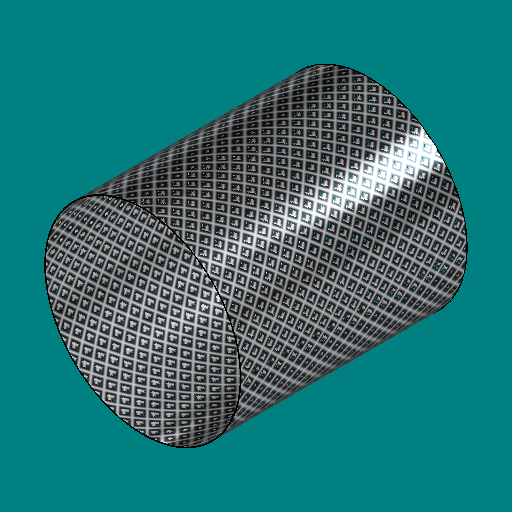
# Autodesk Inventor part: probe-port-mesh
Saved by Autodesk Inventor 2025 (Build 290162000, 162)
## iProperties
Created: 2024-06-28
Part Number: probe-port-mesh
Material: Stainless Steel
Document SubType Name: Modeling
Designer: kuzmin
Density: 8 g/cm^3
Appearance: Expanded Metal 02
Author: kuzmin
Autodesk Inventor part; units mm, degrees
ref_plane "YZ Plane" through (0, 0, 0) normal (1, 0, 0) x (0, 1, 0)
ref_plane "XZ Plane" through (0, 0, 0) normal (0, 1, 0) x (-1, 0, 0)
ref_plane "XY Plane" through (0, 0, 0) normal (0, 0, 1) x (1, 0, 0)
sketch "Sketch1" plane through (0, 0, 0) normal (0, 0, 1) x (1, 0, 0)
  circle A0 centre (0, 0) radius 34.7
  circle A1 centre (0, 0) radius 34.5
  dimension "d0" = 69
  dimension "d1" = 0.2
  constraints: 2 centre point, 2 coincident
  measures "d0" diameter of A1
  measures "d1" radial gap between concentric circles of A1 A0
extrude "Extrusion1" add sketch "Sketch1" along normal blind 80
body "Solid1"
